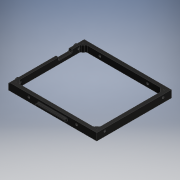
# Autodesk Inventor part: Structure_-Z
Saved by Autodesk Inventor 2018 (Build 220112000, 112)
## iProperties
Created: 2018-07-04
Part Number: Structure_-Z
Material: Aluminum 6061
Document SubType Name: Modeling
Designer: Bradley
Density: 2.7 g/cm^3
Appearance: Anodized - Dark Gray
Mass: 28.4001 g
Surface Area: 88.8306 cm^2
Volume: 10.5186 cm^3
Author: Bradley
Autodesk Inventor part; units mm, degrees
ref_plane "YZ Plane" through (0, 0, 0) normal (1, 0, 0) x (0, 1, 0)
ref_plane "XZ Plane" through (0, 0, 0) normal (0, 1, 0) x (-1, 0, 0)
ref_plane "XY Plane" through (0, 0, 0) normal (0, 0, 1) x (1, 0, 0)
sketch "Sketch1" plane through (0, 0, 0) normal (0, 0, 1) x (1, 0, 0)
  line L0 (49, -41.5) -> (-49, -41.5)
  line L1 (-49, -41.5) -> (-49, 41.5)
  line L2 (-49, 41.5) -> (49, 41.5)
  line L3 (49, 41.5) -> (49, -41.5)
  line L4 (49, -41.5) -> (-49, 41.5) construction
  line L5 (-49, -41.5) -> (49, 41.5) construction
  point P0 (0, 0)
  dimension "d0" = 98
  dimension "d1" = 83
  constraints: 12 end point, 2 midpoint, 2 parallel, 1 horizontal, 1 perpendicular
  measures "d0" distance of L1.end L2.end
  measures "d1" distance of L0.end L1.end
extrude "Extrusion1" add sketch "Sketch1" along normal mid plane 8
sketch "Sketch2" plane through (-49, -41.5, 4) normal (0, -1, 0) x (1, 0, 0)
  line L0 (98, -8) -> (98, 0) projected
  line L1 (0, 0) -> (98, 0) projected
  line L2 (0, 0) -> (0, -8) projected
  line L3 (98, -8) -> (0, -8) projected
  line L4 (34, -4) -> (64, -4) construction
  line L5 (34, -5.5) -> (64, -5.5)
  line L6 (64, -2.5) -> (34, -2.5)
  arc A0 (34, -2.5) -> (34, -5.5) centre (34, -4) ccw
  arc A1 (64, -5.5) -> (64, -2.5) centre (64, -4) ccw
  point P0 (49, -4)
  dimension "d5" = 3
  dimension "d8" = 30
  constraints: 8 end point, 4 point on circle, 4 tangent, 2 centre point, 1 horizontal, 1 midpoint, 1 parallel
  measures "d5" diameter of A1
  measures "d8" distance of L4.start L4.end
extrude "Extrusion2" add sketch "Sketch2" along normal blind 3 contours A0 L6 A1 L5
sketch "Sketch3" plane through (-49, -41.5, 4) normal (0, -1, 0) x (1, 0, 0)
  arc A0 (34, -2.5) -> (34, -5.5) centre (34, -4) ccw projected
  line L0 (34, -2.5) -> (64, -2.5) projected
  arc A1 (64, -5.5) -> (64, -2.5) centre (64, -4) ccw projected
  line L1 (64, -5.5) -> (34, -5.5) projected
  line L2 (98, -8) -> (98, 0) projected
  line L3 (0, 0) -> (98, 0) projected
  line L4 (0, 0) -> (0, -8) projected
  line L5 (98, -8) -> (0, -8) projected
  line L6 (22.5, -3.5) -> (75.5, -3.5) construction
  point P0 (49, -3.5)
  point P1 (49, -8)
  dimension "d9" = 53
  dimension "d39" = 4.5
  constraints: 2 coincident, 2 end point, 2 midpoint, 1 horizontal, 1 vertical alignment
  measures "d9" distance of L6.start L6.end
  measures "d39" distance between parallel lines of L5 L6
hole "Hole1" at (-26.5, -41.5, 0.5) at (26.5, -41.5, 0.5) direction (0, 1, 0) diameter 2.459 depth 5 tip angle 118 thread size "M3x0.5" class "6H" standard "ANSI Metric M Profile"
mirror "Mirror1" about plane through (0, 0, 0) normal (0, 1, 0) of "Extrusion2", "Hole1"
fillet "Fillet1" radius 0.381 8 edges at (16.5, -41.5, 0) (0, -41.5, -1.5) (-16.5, -41.5, 0) (0, -41.5, 1.5) (-16.5, 41.5, 0) (0, 41.5, -1.5) (16.5, 41.5, 0) (0, 41.5, 1.5)
chamfer "Chamfer1" distance 0.5 angle 45 8 edges at (0, -44.5, 1.5) (-16.5, -44.5, 0) (0, -44.5, -1.5) (16.5, -44.5, 0) (0, 44.5, 1.5) (-16.5, 44.5, 0) (0, 44.5, -1.5) (16.5, 44.5, 0)
sketch "Sketch4" plane through (49, -41.5, 4) normal (1, 0, 0) x (0, 0, -1)
  line L0 (3, 9) -> (3, 74) construction
  line L1 (8, 83) -> (8, 0) projected
  line L2 (0, 83) -> (8, 83) projected
  line L3 (8, 0) -> (0, 0) projected
  line L4 (8, 83) -> (8, 0) projected
  line L5 (0, 0) -> (0, 83) projected
  line L6 (0, 0) -> (0, 83) projected
  point P0 (3, 41.5)
  point P1 (4, 41.5)
  dimension "d21" = 65
  dimension "d29" = 5
  constraints: 2 coincident, 2 end point, 1 horizontal alignment, 1 midpoint, 1 vertical
  measures "d21" distance of L0.start L0.end
  measures "d29" distance between parallel lines of L1 L0
hole "Hole2" at (49, -32.5, 1) at (49, 32.5, 1) direction (-1, 0, 0) diameter 2.459 depth 4 tip angle 118 thread size "M3x0.5" class "6H" standard "ANSI Metric M Profile"
mirror "Mirror2" about plane through (0, 0, 0) normal (1, 0, 0) of "Hole2"
sketch "Sketch6" plane through (-49, -41.5, 4) normal (-1, 0, 0) x (0, 0, 1)
  circle A0 centre (-3, 9) radius 1.2295 projected
  circle A1 centre (-3, 74) radius 1.2295 projected
  line L0 (0, 0) -> (-8, 0) projected
  line L1 (0, 83) -> (0, 0) projected
  line L2 (0, 83) -> (-8, 83) projected
  line L3 (-8, 0) -> (-8, 83) projected
  line L4 (-8, 0) -> (0, 0) projected
  arc A2 (-1.1, 71.8091) -> (-1.1, 76.1909) centre (-3, 74) ccw
  arc A3 (-1.1, 6.8091) -> (-1.1, 11.1909) centre (-3, 9) ccw
  line L5 (-1.1, 6.8091) -> (-1.1, 0)
  line L6 (-1.1, 83) -> (-1.1, 76.1909)
  line L7 (-1.1, 71.8091) -> (-1.1, 11.1909)
  point P0 (-4, 41.5)
  dimension "d44" = 1.1
  dimension "d45" = 2.9
  constraints: 6 end point, 4 point on circle, 3 vertical, 2 centre point, 2 collinear, 2 concentric, 2 point on line, 1 equal radius
  measures "d44" distance between parallel lines of L7 L1
  measures "d45" radius of A2
extrude "Extrusion4" cut sketch "Sketch6" against normal blind 1.1 contours L0 L5 A3 L7 A2 L6 L2 L1
sketch "Sketch7" plane through (0, 0, 4) normal (0, 0, 1) x (1, 0, 0)
  line L0 (-47.9, 41.5) -> (-47.9, -41.5) projected
  line L1 (-47.9, -41.5) -> (49, -41.5) projected
  line L2 (49, -41.5) -> (49, 41.5) projected
  line L3 (49, 41.5) -> (-47.9, 41.5) projected
  line L4 (27.7295, 36.5) -> (26.5, 35.7612) projected
  line L5 (25.2705, 36.5) -> (26.5, 35.7612) projected
  line L6 (44.2612, 32.5) -> (45, 33.7295) projected
  line L7 (44.2612, 32.5) -> (45, 31.2705) projected
  line L8 (0, 37.5) -> (0, -37.5) construction
  line L9 (-42, 37.5) -> (42, 37.5)
  line L10 (42, -37.5) -> (-42, -37.5)
  line L11 (45, -34.5) -> (45, 34.5)
  line L12 (-45, 34.5) -> (-45, -34.5)
  arc A0 (-42, -37.5) -> (-45, -34.5) centre (-45, -37.5) ccw
  arc A1 (-45, 34.5) -> (-42, 37.5) centre (-45, 37.5) ccw
  arc A2 (42, 37.5) -> (45, 34.5) centre (45, 37.5) ccw
  arc A3 (45, -34.5) -> (42, -37.5) centre (45, -37.5) ccw
  line L13 (-49, -30.3091) -> (-49, 30.3091) projected
  point P0 (0, 0)
  point P1 (0, 0)
  dimension "d48" = 4
  dimension "d68" = 3
  dimension "d69" = 4
  constraints: 10 end point, 8 line through centre, 8 point on circle, 4 centre point, 3 midpoint, 2 parallel, 2 symmetric about line, 1 coincident, 1 equal radius, 1 horizontal, 1 vertical, 1 other
  measures "d48" distance between parallel lines of L9 L3
  measures "d68" radius of A1
  measures "d69" distance between parallel lines of L12 L13
extrude "Extrusion5" cut sketch "Sketch7" against normal through all contours L7 L11 A3 L10 A0 L12 A1 L9 A2 L6 | L6 L11 L7
sketch "Sketch8" plane through (0, 0, -4) normal (0, 0, -1) x (-1, 0, 0)
  line L0 (-42, 37.5) -> (42, 37.5) projected
  line L1 (42, -37.5) -> (-42, -37.5) projected
  line L2 (-49, -41.5) -> (49, -41.5) projected
  line L3 (49, -41.5) -> (49, 41.5) projected
  line L4 (49, 41.5) -> (-49, 41.5) projected
  line L5 (-49, 41.5) -> (-49, -41.5) projected
  line L6 (45, -40.1) -> (-45, -40.1)
  line L7 (-47.6, -37.5) -> (-47.6, 37.5)
  line L8 (-45, 40.1) -> (45, 40.1)
  line L9 (47.6, 37.5) -> (47.6, -37.5)
  arc A0 (45, -40.1) -> (47.6, -37.5) centre (45, -37.5) ccw
  arc A1 (-47.6, -37.5) -> (-45, -40.1) centre (-45, -37.5) ccw
  arc A2 (-45, 40.1) -> (-47.6, 37.5) centre (-45, 37.5) ccw
  arc A3 (47.6, 37.5) -> (45, 40.1) centre (45, 37.5) ccw
  line L10 (45, 34.5) -> (45, -34.5) projected
  line L11 (-45, -34.5) -> (-45, 34.5) projected
  arc A4 (42, 37.5) -> (45, 34.5) centre (45, 37.5) ccw projected
  arc A5 (45, -34.5) -> (42, -37.5) centre (45, -37.5) ccw projected
  arc A6 (-42, -37.5) -> (-45, -34.5) centre (-45, -37.5) ccw projected
  arc A7 (-45, 34.5) -> (-42, 37.5) centre (-45, 37.5) ccw projected
  point P0 (0, 0)
  dimension "d54" = 1.4
  dimension "d55" = 2.6
  constraints: 8 end point, 8 point on circle, 8 tangent, 4 centre point, 3 equal radius, 3 other
  measures "d54" distance between parallel lines of L6 L2
  measures "d55" radius of A0
extrude "Extrusion6" cut sketch "Sketch8" against normal blind 1 contours L6 A1 L7 A2 L8 A3 L9 A0
sketch "Sketch9" plane through (0, 0, -3) normal (0, 0, -1) x (-1, 0, 0)
  line L0 (42, 37.5) -> (-42, 37.5) projected
  line L1 (45, -34.5) -> (45, 34.5) projected
  line L2 (-42, -37.5) -> (42, -37.5) projected
  line L3 (-45, 34.5) -> (-45, -34.5) projected
  line L4 (45, -40.1) -> (-45, -40.1) projected
  arc A0 (45, -40.1) -> (47.6, -37.5) centre (45, -37.5) ccw projected
  line L5 (47.6, 37.5) -> (47.6, -37.5) projected
  arc A1 (47.6, 37.5) -> (45, 40.1) centre (45, 37.5) ccw projected
  line L6 (-45, 40.1) -> (45, 40.1) projected
  arc A2 (-45, 40.1) -> (-47.6, 37.5) centre (-45, 37.5) ccw projected
  line L7 (-47.6, -37.5) -> (-47.6, 37.5) projected
  arc A3 (-47.6, -37.5) -> (-45, -40.1) centre (-45, -37.5) ccw projected
  arc A4 (-45, 34.5) -> (-42, 37.5) centre (-45, 37.5) ccw projected
  arc A5 (42, 37.5) -> (45, 34.5) centre (45, 37.5) ccw projected
  arc A6 (45, -34.5) -> (42, -37.5) centre (45, -37.5) ccw projected
  arc A7 (-42, -37.5) -> (-45, -34.5) centre (-45, -37.5) ccw projected
  point P0 (0, 0)
  constraints: 4 coincident
hole "Hole3" at (-45, -37.5, -3) at (45, -37.5, -3) at (45, 37.5, -3) at (-45, 37.5, -3) direction (0, 0, 1) diameter 1.567 end through all thread size "M2x0.4" class "6H" standard "ANSI Metric M Profile"
sketch "Sketch11" plane through (0, 0, 4) normal (0, 0, 1) x (1, 0, 0)
  circle A0 centre (45, 37.5) radius 0.7835 projected
  circle A1 centre (-45, -37.5) radius 0.7835 projected
  circle A2 centre (45, -37.5) radius 0.7835 projected
  circle A3 centre (-45, 37.5) radius 0.7835 projected
  arc A4 (-45, 34.5) -> (-42, 37.5) centre (-45, 37.5) ccw projected
  line L0 (-42, 37.5) -> (42, 37.5) projected
  arc A5 (42, 37.5) -> (45, 34.5) centre (45, 37.5) ccw projected
  line L1 (45, 34.5) -> (45, -34.5) projected
  arc A6 (45, -34.5) -> (42, -37.5) centre (45, -37.5) ccw projected
  line L2 (42, -37.5) -> (-42, -37.5) projected
  arc A7 (-42, -37.5) -> (-45, -34.5) centre (-45, -37.5) ccw projected
  line L3 (-45, -34.5) -> (-45, 34.5) projected
  line L4 (-47.9, 41.5) -> (-47.9, -41.5) projected
  line L5 (-47.9, -41.5) -> (49, -41.5) projected
  line L6 (49, -41.5) -> (49, 41.5) projected
  line L7 (49, 41.5) -> (-47.9, 41.5) projected
  line L8 (-49, -30.3091) -> (-49, 30.3091) projected
  line L9 (-49, -30.3091) -> (-47.9, -30.3091) projected
  line L10 (-47.9, -30.3091) -> (-47.9, 30.3091) projected
  line L11 (-49, 30.3091) -> (-47.9, 30.3091) projected
  line L12 (-45, -34.5) -> (-45, 34.5) projected
  line L13 (-45, 25) -> (-49, 25)
  line L14 (-49, 25) -> (-49, 10)
  line L15 (-49, 10) -> (-45, 10)
  line L16 (-45, 10) -> (-45, 25)
  point P0 (0, 0)
  dimension "d70" = 15
  dimension "d71" = 10
  constraints: 8 end point, 2 parallel, 2 point on line, 1 horizontal, 1 perpendicular
  measures "d70" distance between parallel lines of L15 L13
  measures "d71" distance from line of point (0, 0) L15
extrude "Extrusion7" cut sketch "Sketch11" against normal blind 3 contours L3 L15 L4 L13 | L4 L15 L8 L13
fillet "Fillet3" radius 1 6 edges at (-47, 25, 1) (-47, 10, 1) (-48.45, 34.6909, 2.9) (-48.45, 30.3091, 2.9) (-48.45, -30.3091, 2.9) (-48.45, -34.6909, 2.9)
fillet "Fillet3" radius 2 8 edges at (-42, -37.5, 0.5) (-45, -34.5, 0.5) (-45, 34.5, 0.5) (-42, 37.5, 0.5) (45, 34.5, 0.5) (42, 37.5, 0.5) (45, -34.5, 0.5) (42, -37.5, 0.5)
chamfer "Chamfer4" distance 0.5 angle 45 10 edges at (-49, 10.2929, 1.2929) (-49, 10, 2.45) (-49, 17.5, 1) (-49, 24.7071, 1.2929) (-49, 25, 2.45) (-45, 10.2929, 1.2929) (-45, 17.5, 1) (-45, 24.7071, 1.2929) (-45, 25, 3) (-45, 10, 3)
equation "\"d69\" = d48"
body "Solid1"
